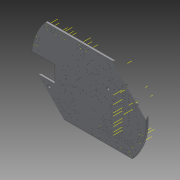
# Autodesk Inventor part: pcb
Saved by Autodesk Inventor 2014 (Build 180170000, 170)
## iProperties
Created: 2013-08-24
Part Number: pcb
Material: Generisch
Document SubType Name: Modeling
Designer: Felix
Density: 1 g/cm^3
Appearance: Vorgabe
Mass: 12.5632 g
Surface Area: 148.317 cm^2
Volume: 12.5632 cm^3
Author: Felix
Autodesk Inventor part; units mm, degrees
ref_plane "YZ Plane" through (0, 0, 0) normal (1, 0, 0) x (0, 1, 0)
ref_plane "XZ Plane" through (0, 0, 0) normal (0, 1, 0) x (-1, 0, 0)
ref_plane "XY Plane" through (0, 0, 0) normal (0, 0, 1) x (1, 0, 0)
sketch "Skizze6" plane through (0, 0, 0) normal (0, 1, 0) x (-1, 0, 0)
  circle A0 centre (10.255, 9.23) radius 0.75
  circle A1 centre (17.67, 60.315) radius 0.75
  circle A2 centre (7.87, 44.425) radius 0.75
  circle A3 centre (17.77, 43.405) radius 0.75
  arc A4 (101.2213, 24.5689) -> (101.2218, 24.5688) centre (101.22155, 24.56885) ccw
  circle A5 centre (77.705, 71.07) radius 0.75
  circle A6 centre (11.055, 72.63) radius 0.75
  circle A7 centre (60.675, 71.27) radius 0.75
  circle A8 centre (78.855, 9.13) radius 0.75
  circle A9 centre (91.045, 71.07) radius 0.75
  circle A10 centre (32.7, 50.6) radius 1.4
  circle A11 centre (87.3, 25.1) radius 1.4
  arc A12 (10.3, 5.7508) -> (10.3, 5.6492) centre (10.3, 5.7) ccw
  arc A13 (91, 5.6492) -> (91, 5.7508) centre (91, 5.7) ccw
  line L0 (10.3, 5.7) -> (91, 5.7)
  arc A14 (10.3, 74.8508) -> (10.3, 74.7492) centre (10.3, 74.8) ccw
  arc A15 (90.6, 74.7492) -> (90.6, 74.8508) centre (90.6, 74.8) ccw
  line L1 (10.3, 74.8) -> (90.6, 74.8)
  arc A16 (91.5301, 73.9834) -> (91.5297, 73.9831) centre (91.5299, 73.98325) ccw
  arc A17 (91.5297, 6.6169) -> (91.5301, 6.6166) centre (91.5299, 6.61675) ccw
  arc A18 (91.5301, 73.9834) -> (91.5297, 73.9831) centre (91.5299, 73.98325) ccw
  arc A19 (101.2213, 24.5689) -> (101.2218, 24.5688) centre (101.22155, 24.56885) ccw
  arc A20 (101.2218, 24.5688) -> (101.2213, 24.5689) centre (101.22155, 24.56885) ccw
  arc A21 (91.5297, 6.6169) -> (91.5301, 6.6166) centre (91.5299, 6.61675) ccw
  arc A22 (91.5299, 6.6167) -> (101.2216, 24.5689) centre (50.590633, 40.310418) ccw
  arc A23 (91.5301, 73.9834) -> (91.5297, 73.9831) centre (91.5299, 73.98325) ccw
  arc A24 (101.2213, 56.0311) -> (101.2218, 56.0312) centre (101.22155, 56.03115) ccw
  arc A25 (101.2216, 56.0312) -> (91.5299, 73.9833) centre (50.590888, 40.289632) ccw
  arc A26 (101.2218, 56.0312) -> (101.2213, 56.0311) centre (101.22155, 56.03115) ccw
  arc A27 (101.2213, 24.5689) -> (101.2218, 24.5688) centre (101.22155, 24.56885) ccw
  arc A28 (91.5301, 73.9834) -> (91.5297, 73.9831) centre (91.5299, 73.98325) ccw
  arc A29 (101.2213, 56.0311) -> (101.2218, 56.0312) centre (101.22155, 56.03115) ccw
  arc A30 (101.2216, 56.0312) -> (91.5299, 73.9833) centre (50.590888, 40.289632) ccw
  arc A31 (101.2218, 56.0312) -> (101.2213, 56.0311) centre (101.22155, 56.03115) ccw
  arc A32 (101.2213, 24.5689) -> (101.2218, 24.5688) centre (101.22155, 24.56885) ccw
  arc A33 (101.2218, 24.5688) -> (101.2213, 24.5689) centre (101.22155, 24.56885) ccw
  arc A34 (91.5297, 6.6169) -> (91.5301, 6.6166) centre (91.5299, 6.61675) ccw
  arc A35 (91.5299, 6.6167) -> (101.2216, 24.5689) centre (50.590633, 40.310418) ccw
  arc A36 (91.5301, 73.9834) -> (91.5297, 73.9831) centre (91.5299, 73.98325) ccw
  arc A37 (101.2213, 56.0311) -> (101.2218, 56.0312) centre (101.22155, 56.03115) ccw
  arc A38 (101.2216, 56.0312) -> (91.5299, 73.9833) centre (50.590888, 40.289632) ccw
  arc A39 (101.2218, 56.0312) -> (101.2213, 56.0311) centre (101.22155, 56.03115) ccw
  arc A40 (101.2213, 24.5689) -> (101.2218, 24.5688) centre (101.22155, 24.56885) ccw
  arc A41 (101.2218, 24.5688) -> (101.2213, 24.5689) centre (101.22155, 24.56885) ccw
  arc A42 (91.5297, 6.6169) -> (91.5301, 6.6166) centre (91.5299, 6.61675) ccw
  arc A43 (91.5299, 6.6167) -> (101.2216, 24.5689) centre (50.590633, 40.310418) ccw
  arc A44 (91.5301, 73.9834) -> (91.5297, 73.9831) centre (91.5299, 73.98325) ccw
  arc A45 (101.2213, 56.0311) -> (101.2218, 56.0312) centre (101.22155, 56.03115) ccw
  arc A46 (101.2216, 56.0312) -> (91.5299, 73.9833) centre (50.590888, 40.289632) ccw
  arc A47 (101.2218, 56.0312) -> (101.2213, 56.0311) centre (101.22155, 56.03115) ccw
  arc A48 (101.2213, 24.5689) -> (101.2218, 24.5688) centre (101.22155, 24.56885) ccw
  arc A49 (101.2218, 24.5688) -> (101.2213, 24.5689) centre (101.22155, 24.56885) ccw
  arc A50 (91.5297, 6.6169) -> (91.5301, 6.6166) centre (91.5299, 6.61675) ccw
  arc A51 (91.5299, 6.6167) -> (101.2216, 24.5689) centre (50.590633, 40.310418) ccw
  arc A52 (91.5301, 73.9834) -> (91.5297, 73.9831) centre (91.5299, 73.98325) ccw
  arc A53 (101.2213, 56.0311) -> (101.2218, 56.0312) centre (101.22155, 56.03115) ccw
  arc A54 (101.2216, 56.0312) -> (91.5299, 73.9833) centre (50.590888, 40.289632) ccw
  arc A55 (101.2218, 56.0312) -> (101.2213, 56.0311) centre (101.22155, 56.03115) ccw
  arc A56 (101.2213, 24.5689) -> (101.2218, 24.5688) centre (101.22155, 24.56885) ccw
  arc A57 (101.2218, 24.5688) -> (101.2213, 24.5689) centre (101.22155, 24.56885) ccw
  arc A58 (91.5297, 6.6169) -> (91.5301, 6.6166) centre (91.5299, 6.61675) ccw
  arc A59 (91.5299, 6.6167) -> (101.2216, 24.5689) centre (50.590633, 40.310418) ccw
  arc A60 (98.4945, 63.0178) -> (98.4941, 63.0176) centre (98.4943, 63.0177) ccw
  arc A61 (101.2213, 56.0311) -> (101.2218, 56.0312) centre (101.22155, 56.03115) ccw
  arc A62 (101.2216, 56.0312) -> (98.4943, 63.0177) centre (50.580091, 40.287993) ccw
  arc A63 (91.5301, 73.9834) -> (91.5297, 73.9831) centre (91.5299, 73.98325) ccw
  arc A64 (98.4941, 63.0176) -> (98.4945, 63.0178) centre (98.4943, 63.0177) ccw
  arc A65 (98.4943, 63.0177) -> (91.5299, 73.9833) centre (50.605086, 40.297009) ccw
  arc A66 (98.4945, 63.0178) -> (98.4941, 63.0176) centre (98.4943, 63.0177) ccw
  arc A67 (101.2213, 56.0311) -> (101.2218, 56.0312) centre (101.22155, 56.03115) ccw
  arc A68 (101.2216, 56.0312) -> (98.4943, 63.0177) centre (50.580091, 40.287993) ccw
  arc A69 (101.2218, 56.0312) -> (101.2213, 56.0311) centre (101.22155, 56.03115) ccw
  arc A70 (101.2213, 24.5689) -> (101.2218, 24.5688) centre (101.22155, 24.56885) ccw
  arc A71 (101.2218, 24.5688) -> (101.2213, 24.5689) centre (101.22155, 24.56885) ccw
  arc A72 (91.5297, 6.6169) -> (91.5301, 6.6166) centre (91.5299, 6.61675) ccw
  arc A73 (91.5299, 6.6167) -> (101.2216, 24.5689) centre (50.590633, 40.310418) ccw
  arc A74 (9.6899, 6.6166) -> (9.6903, 6.6169) centre (9.6901, 6.61675) ccw
  arc A75 (9.6903, 73.9831) -> (9.6899, 73.9834) centre (9.6901, 73.98325) ccw
  arc A76 (9.6901, 73.9833) -> (9.6901, 6.6167) centre (50.615687, 40.3) ccw
  arc A77 (9.6899, 6.6166) -> (9.6903, 6.6169) centre (9.6901, 6.61675) ccw
  arc A78 (9.6903, 73.9831) -> (9.6899, 73.9834) centre (9.6901, 73.98325) ccw
  arc A79 (9.6901, 73.9833) -> (9.6901, 6.6167) centre (50.615687, 40.3) ccw
  arc A80 (9.6899, 6.6166) -> (9.6903, 6.6169) centre (9.6901, 6.61675) ccw
  arc A81 (9.6903, 73.9831) -> (9.6899, 73.9834) centre (9.6901, 73.98325) ccw
  arc A82 (9.6901, 73.9833) -> (9.6901, 6.6167) centre (50.615687, 40.3) ccw
  arc A83 (9.6899, 6.6166) -> (9.6903, 6.6169) centre (9.6901, 6.61675) ccw
  arc A84 (9.6903, 73.9831) -> (9.6899, 73.9834) centre (9.6901, 73.98325) ccw
  arc A85 (9.6901, 73.9833) -> (9.6901, 6.6167) centre (50.615687, 40.3) ccw
  arc A86 (9.6899, 6.6166) -> (9.6903, 6.6169) centre (9.6901, 6.61675) ccw
  arc A87 (9.6903, 73.9831) -> (9.6899, 73.9834) centre (9.6901, 73.98325) ccw
  arc A88 (9.6901, 73.9833) -> (9.6901, 6.6167) centre (50.615687, 40.3) ccw
  arc A89 (9.6899, 6.6166) -> (9.6903, 6.6169) centre (9.6901, 6.61675) ccw
  arc A90 (9.6903, 73.9831) -> (9.6899, 73.9834) centre (9.6901, 73.98325) ccw
  arc A91 (9.6901, 73.9833) -> (9.6901, 6.6167) centre (50.615687, 40.3) ccw
  arc A92 (9.6899, 6.6166) -> (9.6903, 6.6169) centre (9.6901, 6.61675) ccw
  arc A93 (9.6903, 73.9831) -> (9.6899, 73.9834) centre (9.6901, 73.98325) ccw
  arc A94 (9.6901, 73.9833) -> (9.6901, 6.6167) centre (50.615687, 40.3) ccw
  arc A95 (9.6899, 6.6166) -> (9.6903, 6.6169) centre (9.6901, 6.61675) ccw
  arc A96 (9.6903, 73.9831) -> (9.6899, 73.9834) centre (9.6901, 73.98325) ccw
  arc A97 (9.6901, 73.9833) -> (9.6901, 6.6167) centre (50.615687, 40.3) ccw
  arc A98 (9.6899, 6.6166) -> (9.6903, 6.6169) centre (9.6901, 6.61675) ccw
  arc A99 (9.6903, 73.9831) -> (9.6899, 73.9834) centre (9.6901, 73.98325) ccw
  arc A100 (9.6901, 73.9833) -> (9.6901, 6.6167) centre (50.615687, 40.3) ccw
  arc A101 (91.5301, 73.9834) -> (91.5297, 73.9831) centre (91.5299, 73.98325) ccw
  arc A102 (98.4941, 63.0176) -> (98.4945, 63.0178) centre (98.4943, 63.0177) ccw
  arc A103 (98.4943, 63.0177) -> (91.5299, 73.9833) centre (50.605086, 40.297009) ccw
  arc A104 (98.4945, 63.0178) -> (98.4941, 63.0176) centre (98.4943, 63.0177) ccw
  arc A105 (101.2213, 56.0311) -> (101.2218, 56.0312) centre (101.22155, 56.03115) ccw
  arc A106 (101.2216, 56.0312) -> (98.4943, 63.0177) centre (50.580091, 40.287993) ccw
  arc A107 (101.2218, 56.0312) -> (101.2213, 56.0311) centre (101.22155, 56.03115) ccw
  arc A108 (101.2218, 24.5688) -> (101.2213, 24.5689) centre (101.22155, 24.56885) ccw
  arc A109 (91.5297, 6.6169) -> (91.5301, 6.6166) centre (91.5299, 6.61675) ccw
  arc A110 (91.5299, 6.6167) -> (101.2216, 24.5689) centre (50.590633, 40.310418) ccw
  arc A111 (91.5301, 73.9834) -> (91.5297, 73.9831) centre (91.5299, 73.98325) ccw
  arc A112 (98.4941, 63.0176) -> (98.4945, 63.0178) centre (98.4943, 63.0177) ccw
  arc A113 (98.4943, 63.0177) -> (91.5299, 73.9833) centre (50.605086, 40.297009) ccw
  arc A114 (98.4945, 63.0178) -> (98.4941, 63.0176) centre (98.4943, 63.0177) ccw
  arc A115 (101.2213, 56.0311) -> (101.2218, 56.0312) centre (101.22155, 56.03115) ccw
  arc A116 (101.2216, 56.0312) -> (98.4943, 63.0177) centre (50.580091, 40.287993) ccw
  arc A117 (101.2218, 56.0312) -> (101.2213, 56.0311) centre (101.22155, 56.03115) ccw
  arc A118 (101.2213, 24.5689) -> (101.2218, 24.5688) centre (101.22155, 24.56885) ccw
  arc A119 (101.2218, 24.5688) -> (101.2213, 24.5689) centre (101.22155, 24.56885) ccw
  arc A120 (91.5297, 6.6169) -> (91.5301, 6.6166) centre (91.5299, 6.61675) ccw
  arc A121 (91.5299, 6.6167) -> (101.2216, 24.5689) centre (50.590633, 40.310418) ccw
  arc A122 (98.4945, 63.0178) -> (98.4941, 63.0176) centre (98.4943, 63.0177) ccw
  arc A123 (101.2213, 56.0311) -> (101.2218, 56.0312) centre (101.22155, 56.03115) ccw
  arc A124 (101.2216, 56.0312) -> (98.4943, 63.0177) centre (50.580091, 40.287993) ccw
  arc A125 (91.5301, 73.9834) -> (91.5297, 73.9831) centre (91.5299, 73.98325) ccw
  arc A126 (98.4941, 63.0176) -> (98.4945, 63.0178) centre (98.4943, 63.0177) ccw
  arc A127 (98.4943, 63.0177) -> (91.5299, 73.9833) centre (50.605086, 40.297009) ccw
  arc A128 (98.4945, 63.0178) -> (98.4941, 63.0176) centre (98.4943, 63.0177) ccw
  arc A129 (101.2213, 56.0311) -> (101.2218, 56.0312) centre (101.22155, 56.03115) ccw
  arc A130 (101.2216, 56.0312) -> (98.4943, 63.0177) centre (50.580091, 40.287993) ccw
  arc A131 (101.2218, 56.0312) -> (101.2213, 56.0311) centre (101.22155, 56.03115) ccw
  arc A132 (98.4941, 17.5824) -> (98.4945, 17.5822) centre (98.4943, 17.5823) ccw
  arc A133 (98.4945, 17.5822) -> (98.4941, 17.5824) centre (98.4943, 17.5823) ccw
  arc A134 (91.5297, 6.6169) -> (91.5301, 6.6166) centre (91.5299, 6.61675) ccw
  arc A135 (91.5299, 6.6167) -> (98.4943, 17.5823) centre (50.605086, 40.302991) ccw
  arc A136 (91.5301, 73.9834) -> (91.5297, 73.9831) centre (91.5299, 73.98325) ccw
  arc A137 (98.4941, 63.0176) -> (98.4945, 63.0178) centre (98.4943, 63.0177) ccw
  arc A138 (98.4943, 63.0177) -> (91.5299, 73.9833) centre (50.605086, 40.297009) ccw
  arc A139 (98.4945, 63.0178) -> (98.4941, 63.0176) centre (98.4943, 63.0177) ccw
  arc A140 (101.2213, 56.0311) -> (101.2218, 56.0312) centre (101.22155, 56.03115) ccw
  arc A141 (101.2216, 56.0312) -> (98.4943, 63.0177) centre (50.580091, 40.287993) ccw
  arc A142 (101.2218, 56.0312) -> (101.2213, 56.0311) centre (101.22155, 56.03115) ccw
  arc A143 (98.4941, 17.5824) -> (98.4945, 17.5822) centre (98.4943, 17.5823) ccw
  arc A144 (98.4945, 17.5822) -> (98.4941, 17.5824) centre (98.4943, 17.5823) ccw
  arc A145 (91.5297, 6.6169) -> (91.5301, 6.6166) centre (91.5299, 6.61675) ccw
  arc A146 (91.5299, 6.6167) -> (98.4943, 17.5823) centre (50.605086, 40.302991) ccw
  arc A147 (91.5301, 73.9834) -> (91.5297, 73.9831) centre (91.5299, 73.98325) ccw
  arc A148 (98.4941, 63.0176) -> (98.4945, 63.0178) centre (98.4943, 63.0177) ccw
  arc A149 (98.4943, 63.0177) -> (91.5299, 73.9833) centre (50.605086, 40.297009) ccw
  arc A150 (98.4945, 63.0178) -> (98.4941, 63.0176) centre (98.4943, 63.0177) ccw
  arc A151 (101.2213, 56.0311) -> (101.2218, 56.0312) centre (101.22155, 56.03115) ccw
  arc A152 (101.2216, 56.0312) -> (98.4943, 63.0177) centre (50.580091, 40.287993) ccw
  arc A153 (101.2218, 56.0312) -> (101.2213, 56.0311) centre (101.22155, 56.03115) ccw
  arc A154 (98.4941, 17.5824) -> (98.4945, 17.5822) centre (98.4943, 17.5823) ccw
  arc A155 (98.4945, 17.5822) -> (98.4941, 17.5824) centre (98.4943, 17.5823) ccw
  arc A156 (91.5297, 6.6169) -> (91.5301, 6.6166) centre (91.5299, 6.61675) ccw
  arc A157 (91.5299, 6.6167) -> (98.4943, 17.5823) centre (50.605086, 40.302991) ccw
  arc A158 (91.5301, 73.9834) -> (91.5297, 73.9831) centre (91.5299, 73.98325) ccw
  arc A159 (98.4941, 63.0176) -> (98.4945, 63.0178) centre (98.4943, 63.0177) ccw
  arc A160 (98.4943, 63.0177) -> (91.5299, 73.9833) centre (50.605086, 40.297009) ccw
  arc A161 (98.4945, 63.0178) -> (98.4941, 63.0176) centre (98.4943, 63.0177) ccw
  arc A162 (101.2213, 56.0311) -> (101.2218, 56.0312) centre (101.22155, 56.03115) ccw
  arc A163 (101.2216, 56.0312) -> (98.4943, 63.0177) centre (50.580091, 40.287993) ccw
  arc A164 (101.2218, 56.0312) -> (101.2213, 56.0311) centre (101.22155, 56.03115) ccw
  arc A165 (98.4941, 17.5824) -> (98.4945, 17.5822) centre (98.4943, 17.5823) ccw
  arc A166 (98.4945, 17.5822) -> (98.4941, 17.5824) centre (98.4943, 17.5823) ccw
  arc A167 (91.5297, 6.6169) -> (91.5301, 6.6166) centre (91.5299, 6.61675) ccw
  arc A168 (91.5299, 6.6167) -> (98.4943, 17.5823) centre (50.605086, 40.302991) ccw
  circle A169 centre (10.4, 20.5) radius 0.254
  circle A170 centre (23.03, 70.23) radius 0.254
  circle A171 centre (31.4, 70.3) radius 0.254
  circle A172 centre (40.4, 42.8) radius 0.254
  circle A173 centre (22.7, 43.5) radius 0.254
  circle A174 centre (20, 45) radius 0.254
  circle A175 centre (58.2, 64.5) radius 0.254
  circle A176 centre (65.6, 60.7) radius 0.254
  circle A177 centre (55.6, 63.3) radius 0.254
  circle A178 centre (46.2, 27.8) radius 0.254
  circle A179 centre (42.8, 57) radius 0.254
  circle A180 centre (61, 69.2) radius 0.254
  circle A181 centre (50.1, 53.6) radius 0.254
  circle A182 centre (52.4, 53.6) radius 0.254
  circle A183 centre (41.2, 60) radius 0.254
  circle A184 centre (48.8, 39.9) radius 0.254
  circle A185 centre (44.1, 39.8) radius 0.254
  circle A186 centre (30.1, 39.4) radius 0.254
  circle A187 centre (37.1, 13.3) radius 0.254
  circle A188 centre (33.2, 13.3) radius 0.254
  circle A189 centre (76.305, 72.87) radius 0.4064
  circle A190 centre (75.035, 70.33) radius 0.4064
  circle A191 centre (73.765, 72.87) radius 0.4064
  circle A192 centre (72.495, 70.33) radius 0.4064
  circle A193 centre (19.57, 42.005) radius 0.4064
  circle A194 centre (17.03, 40.735) radius 0.4064
  circle A195 centre (19.57, 39.465) radius 0.4064
  circle A196 centre (17.03, 38.195) radius 0.4064
  circle A197 centre (19.47, 58.915) radius 0.4064
  circle A198 centre (16.93, 57.645) radius 0.4064
  circle A199 centre (19.47, 56.375) radius 0.4064
  circle A200 centre (16.93, 55.105) radius 0.4064
  circle A201 centre (19.47, 53.835) radius 0.4064
  circle A202 centre (16.93, 52.565) radius 0.4064
  circle A203 centre (19.47, 51.295) radius 0.4064
  circle A204 centre (16.93, 50.025) radius 0.4064
  circle A205 centre (19.47, 48.755) radius 0.4064
  circle A206 centre (16.93, 47.485) radius 0.4064
  circle A207 centre (9.67, 45.825) radius 0.4064
  circle A208 centre (7.13, 47.095) radius 0.4064
  circle A209 centre (9.67, 48.365) radius 0.4064
  circle A210 centre (7.13, 49.635) radius 0.4064
  circle A211 centre (9.67, 50.905) radius 0.4064
  circle A212 centre (7.13, 52.175) radius 0.4064
  circle A213 centre (12.455, 70.83) radius 0.4064
  circle A214 centre (13.725, 73.37) radius 0.4064
  circle A215 centre (14.995, 70.83) radius 0.4064
  circle A216 centre (16.265, 73.37) radius 0.4064
  circle A217 centre (17.535, 70.83) radius 0.4064
  circle A218 centre (18.805, 73.37) radius 0.4064
  circle A219 centre (20.075, 70.83) radius 0.4064
  circle A220 centre (21.345, 73.37) radius 0.4064
  circle A221 centre (11.655, 7.43) radius 0.4064
  circle A222 centre (12.925, 9.97) radius 0.4064
  circle A223 centre (14.195, 7.43) radius 0.4064
  circle A224 centre (15.465, 9.97) radius 0.4064
  circle A225 centre (16.735, 7.43) radius 0.4064
  circle A226 centre (18.005, 9.97) radius 0.4064
  circle A227 centre (19.275, 7.43) radius 0.4064
  circle A228 centre (20.545, 9.97) radius 0.4064
  circle A229 centre (4.9078, 62.6827) radius 0.4064
  circle A230 centre (6.7307, 60.5053) radius 0.4064
  circle A231 centre (3.895, 60.3534) radius 0.4064
  circle A232 centre (5.7179, 58.1759) radius 0.4064
  circle A233 centre (2.8821, 58.0241) radius 0.4064
  circle A234 centre (4.705, 55.8466) radius 0.4064
  circle A235 centre (1.8693, 55.6947) radius 0.4064
  circle A236 centre (3.6922, 53.5173) radius 0.4064
  circle A237 centre (0.3852, 29.2123) radius 0.4064
  circle A238 centre (3.1969, 28.8139) radius 0.4064
  circle A239 centre (1.1912, 26.8036) radius 0.4064
  circle A240 centre (4.0029, 26.4052) radius 0.4064
  circle A241 centre (1.9971, 24.3948) radius 0.4064
  circle A242 centre (4.8088, 23.9964) radius 0.4064
  circle A243 centre (2.8031, 21.9861) radius 0.4064
  circle A244 centre (5.6148, 21.5877) radius 0.4064
  circle A245 centre (59.275, 73.07) radius 0.4064
  circle A246 centre (64.6, 17.4) radius 0.254
  circle A247 centre (56.735, 73.07) radius 0.4064
  circle A248 centre (55.465, 70.53) radius 0.4064
  circle A249 centre (54.195, 73.07) radius 0.4064
  circle A250 centre (52.925, 70.53) radius 0.4064
  circle A251 centre (60.3, 44.5) radius 0.254
  circle A252 centre (80.255, 7.33) radius 0.4064
  circle A253 centre (81.525, 9.87) radius 0.4064
  circle A254 centre (82.795, 7.33) radius 0.4064
  circle A255 centre (84.065, 9.87) radius 0.4064
  circle A256 centre (85.335, 7.33) radius 0.4064
  circle A257 centre (86.605, 9.87) radius 0.4064
  circle A258 centre (87.875, 7.33) radius 0.4064
  circle A259 centre (89.145, 9.87) radius 0.4064
  circle A260 centre (64, 36.4) radius 0.254
  circle A261 centre (89.645, 72.87) radius 0.4064
  circle A262 centre (88.375, 70.33) radius 0.4064
  circle A263 centre (87.105, 72.87) radius 0.4064
  circle A264 centre (85.835, 70.33) radius 0.4064
  circle A265 centre (84.565, 72.87) radius 0.4064
  circle A266 centre (83.295, 70.33) radius 0.4064
  circle A267 centre (82.025, 72.87) radius 0.4064
  circle A268 centre (80.755, 70.33) radius 0.4064
  circle A269 centre (71.9, 28.8) radius 0.254
  circle A270 centre (96.5044, 17.5038) radius 0.4064
  circle A271 centre (94.6288, 19.6361) radius 0.4064
  circle A272 centre (97.46, 19.8572) radius 0.4064
  circle A273 centre (95.5844, 21.9895) radius 0.4064
  circle A274 centre (98.4156, 22.2105) radius 0.4064
  circle A275 centre (96.54, 24.3428) radius 0.4064
  circle A276 centre (99.3712, 24.5639) radius 0.4064
  circle A277 centre (97.4956, 26.6962) radius 0.4064
  circle A278 centre (101.1281, 52.2968) radius 0.4064
  circle A279 centre (98.315, 52.6854) radius 0.4064
  circle A280 centre (100.3137, 54.7027) radius 0.4064
  circle A281 centre (97.5006, 55.0913) radius 0.4064
  circle A282 centre (99.4994, 57.1087) radius 0.4064
  circle A283 centre (96.6863, 57.4973) radius 0.4064
  circle A284 centre (98.685, 59.5146) radius 0.4064
  circle A285 centre (95.8719, 59.9032) radius 0.4064
  circle A286 centre (59.2, 45.4) radius 0.254
  circle A287 centre (62.7, 37) radius 0.254
  circle A288 centre (40.6488, 11.4606) radius 0.508
  circle A289 centre (47.1512, 11.4606) radius 0.508
  circle A290 centre (40.6488, 6.9394) radius 0.508
  circle A291 centre (47.1512, 6.9394) radius 0.508
  circle A292 centre (60.2, 55.087) radius 0.4064
  circle A293 centre (60.2, 59.913) radius 0.4064
  circle A294 centre (19.43, 33.62) radius 0.508
  circle A295 centre (19.43, 31.08) radius 0.508
  circle A296 centre (19.47, 21.59) radius 0.508
  circle A297 centre (19.47, 24.13) radius 0.508
  circle A298 centre (19.47, 26.67) radius 0.508
  circle A299 centre (35.032, 15.304) radius 0.508
  circle A300 centre (29.952, 15.304) radius 0.508
  circle A301 centre (27.412, 15.304) radius 0.508
  circle A302 centre (27.412, 17.844) radius 0.508
  circle A303 centre (24.872, 17.844) radius 0.508
  circle A304 centre (22.332, 15.304) radius 0.508
  circle A305 centre (22.332, 17.844) radius 0.508
  circle A306 centre (19.792, 15.304) radius 0.508
  circle A307 centre (17.252, 15.304) radius 0.508
  circle A308 centre (37.572, 17.844) radius 0.508
  circle A309 centre (32.492, 17.844) radius 0.508
  circle A310 centre (35.032, 17.844) radius 0.508
  circle A311 centre (37.572, 15.304) radius 0.508
  circle A312 centre (40.112, 15.304) radius 0.508
  circle A313 centre (17.252, 17.844) radius 0.508
  circle A314 centre (14.712, 17.844) radius 0.508
  circle A315 centre (12.172, 17.844) radius 0.508
  circle A316 centre (32.492, 15.304) radius 0.508
  circle A317 centre (24.872, 15.304) radius 0.508
  circle A318 centre (14.712, 15.304) radius 0.508
  circle A319 centre (40.112, 17.844) radius 0.508
  circle A320 centre (19.792, 17.844) radius 0.508
  circle A321 centre (12.172, 15.304) radius 0.508
  circle A322 centre (9.632, 15.304) radius 0.508
  circle A323 centre (29.952, 17.844) radius 0.508
  circle A324 centre (9.632, 17.844) radius 0.508
  circle A325 centre (13.4, 54.57) radius 0.508
  circle A326 centre (13.4, 44.41) radius 0.508
  circle A327 centre (13.4, 46.95) radius 0.508
  circle A328 centre (13.4, 34.25) radius 0.508
  circle A329 centre (13.4, 31.71) radius 0.508
  circle A330 centre (13.4, 41.87) radius 0.508
  circle A331 centre (13.4, 36.79) radius 0.508
  circle A332 centre (13.4, 49.49) radius 0.508
  circle A333 centre (13.4, 39.33) radius 0.508
  circle A334 centre (13.4, 52.03) radius 0.508
  circle A335 centre (67.5, 21.8) radius 0.254
  circle A336 centre (29.3, 57.4) radius 0.254
  circle A337 centre (25.4, 47.4) radius 0.254
  circle A338 centre (30.4, 58.3) radius 0.254
  circle A339 centre (26.6, 44.3) radius 0.254
  circle A340 centre (27.1, 52.8) radius 0.254
  circle A341 centre (27.4, 43.2) radius 0.254
  circle A342 centre (27, 40) radius 0.254
  circle A343 centre (29.2, 25.3) radius 0.254
  circle A344 centre (36.9, 52.1) radius 0.254
  circle A345 centre (36, 42.7) radius 0.254
  circle A346 centre (29.7, 32.3) radius 0.254
  circle A347 centre (29.8, 27.1) radius 0.254
  circle A348 centre (32.9, 25.7) radius 0.254
  circle A349 centre (36.5, 57.8) radius 0.254
  circle A350 centre (41.7, 37.3) radius 0.254
  circle A351 centre (42.4, 39.8) radius 0.254
  circle A352 centre (42, 14.1) radius 0.254
  circle A353 centre (51.8, 60.7) radius 0.254
  circle A354 centre (52.1, 55.5) radius 0.254
  circle A355 centre (52.9, 56.8) radius 0.254
  circle A356 centre (55.6, 64.7) radius 0.254
  circle A357 centre (54.6, 67.8) radius 0.254
  circle A358 centre (73.4, 19.4) radius 0.254
  circle A359 centre (78.1, 19.4) radius 0.254
  circle A360 centre (77.4, 16.7) radius 0.254
  circle A361 centre (69.7, 16.8) radius 0.254
  circle A362 centre (77.3, 24.7) radius 0.254
  circle A363 centre (72.9, 27.3) radius 0.254
  circle A364 centre (26.8, 57.4) radius 0.254
  circle A365 centre (30.1, 38) radius 0.254
  circle A366 centre (31.6, 59.4) radius 0.254
  circle A367 centre (27.7, 33) radius 0.254
  circle A368 centre (28.8, 43.2) radius 0.254
  circle A369 centre (30.3, 34.6) radius 0.254
  circle A370 centre (34, 41.7) radius 0.254
  circle A371 centre (32.2, 57.4) radius 0.254
  circle A372 centre (70.6, 42.4) radius 0.254
  circle A373 centre (24.5, 72.5) radius 0.254
  circle A374 centre (71.1, 39.3) radius 0.254
  circle A375 centre (11.2, 60.8) radius 0.254
  circle A376 centre (22.2, 27.1) radius 0.254
  circle A377 centre (72.3, 38.7) radius 0.254
  circle A378 centre (38.7, 23.6) radius 0.254
  circle A379 centre (76, 14.9) radius 0.254
  circle A380 centre (34, 19.5) radius 0.254
  circle A381 centre (75.2, 44) radius 0.254
  circle A382 centre (76.7, 10.1) radius 0.254
  circle A383 centre (10.5, 64.9) radius 0.254
  circle A384 centre (4.7, 37.2) radius 0.254
  circle A385 centre (92.4, 26.6) radius 0.254
  circle A386 centre (62.5, 17.2) radius 0.254
  circle A387 centre (82.8, 17.4) radius 0.254
  circle A388 centre (67.8, 12.5) radius 0.254
  circle A389 centre (37.3, 21) radius 0.254
  circle A390 centre (82.7, 11.6) radius 0.254
  circle A391 centre (8.4, 63) radius 0.254
  circle A392 centre (30, 65.2) radius 0.254
  circle A393 centre (43.5, 43.1) radius 0.254
  circle A394 centre (5.7, 35.9) radius 0.254
  circle A395 centre (7.5, 13.7) radius 0.254
  circle A396 centre (36.7, 23.3) radius 0.254
  circle A397 centre (3.3, 30.6) radius 0.254
  circle A398 centre (69.1, 12.5) radius 0.254
  circle A399 centre (90.2, 17.7) radius 0.254
  circle A400 centre (13.1, 67.2) radius 0.254
  circle A401 centre (11.7, 68.6) radius 0.254
  circle A402 centre (31, 67.1) radius 0.254
  circle A403 centre (43.6, 44.9) radius 0.254
  circle A404 centre (11.5, 12.1) radius 0.254
  circle A405 centre (70, 9) radius 0.254
  circle A406 centre (35.2, 22.6) radius 0.254
  circle A407 centre (90.1, 19.2) radius 0.254
  circle A408 centre (63.5, 15.5) radius 0.254
  circle A409 centre (14.7, 68.1) radius 0.254
  circle A410 centre (29.86, 68.94) radius 0.254
  circle A411 centre (42, 45) radius 0.254
  circle A412 centre (56, 36.9) radius 0.254
  circle A413 centre (37, 26.4) radius 0.254
  circle A414 centre (31.4, 25.7) radius 0.254
  circle A415 centre (63.5, 21.7) radius 0.254
  circle A416 centre (11.2, 59.3) radius 0.254
  circle A417 centre (23.7, 27.1) radius 0.254
  circle A418 centre (64.7, 24.4) radius 0.254
  circle A419 centre (35.6, 24.7) radius 0.254
  circle A420 centre (30.6, 23.7) radius 0.254
  circle A421 centre (65.5, 26.3) radius 0.254
  circle A422 centre (66.6, 29.3) radius 0.254
  circle A423 centre (79.7, 15.9) radius 0.254
  circle A424 centre (67.7, 30.3) radius 0.254
  circle A425 centre (97.8, 48.7) radius 0.254
  circle A426 centre (76.2, 31.4) radius 0.254
  circle A427 centre (74.1, 33.1) radius 0.254
  circle A428 centre (32.9, 70.3) radius 0.254
  circle A429 centre (26.85, 36.1) radius 0.254
  circle A430 centre (31.7, 12.5) radius 0.254
  circle A431 centre (12.6, 63.9) radius 0.254
  circle A432 centre (67.7, 48.9) radius 0.254
  circle A433 centre (95.9, 49.8) radius 0.254
  circle A434 centre (61.3, 37.9) radius 0.254
  circle A435 centre (62.9, 26.4) radius 0.254
  circle A436 centre (62.4, 47.4) radius 0.254
  circle A437 centre (73.5, 12.3) radius 0.254
  circle A438 centre (48.4, 36.7) radius 0.254
  circle A439 centre (68.9, 35.1) radius 0.254
  circle A440 centre (77.5, 33.9) radius 0.254
  circle A441 centre (43.8, 51.3) radius 0.254
  circle A442 centre (41.5, 57.7) radius 0.254
  circle A443 centre (58.5, 34.2) radius 0.254
  circle A444 centre (39.1, 36.7) radius 0.254
  circle A445 centre (52.7, 36.7) radius 0.254
  circle A446 centre (51.1, 72.8) radius 0.254
  circle A447 centre (31.8, 73.1) radius 0.254
  circle A448 centre (49, 45) radius 0.254
  circle A449 centre (42.2, 49.9) radius 0.254
  circle A450 centre (58.005, 70.53) radius 0.4064
  circle A451 centre (66.8, 10.8) radius 0.254
  circle A452 centre (85.4, 13.4) radius 0.254
  circle A453 centre (21.8, 20.7) radius 0.254
  circle A454 centre (30.2, 36.3) radius 0.254
  circle A455 centre (61.1, 11.6) radius 0.254
  circle A456 centre (34, 8.5) radius 0.254
  circle A457 centre (67.9, 73.5) radius 0.254
  circle A458 centre (42, 72.7) radius 0.254
  circle A459 centre (31.8, 68.1) radius 0.254
  circle A460 centre (44.9, 43.2) radius 0.254
  circle A461 centre (29.6, 29.9) radius 0.254
  circle A462 centre (16.7, 29.4) radius 0.254
  circle A463 centre (12.7, 24.2) radius 0.254
  circle A464 centre (61.3, 43.4) radius 0.254
  circle A465 centre (65, 35.6) radius 0.254
  circle A466 centre (72.1, 30.3) radius 0.254
  circle A467 centre (59, 51) radius 0.254
  circle A468 centre (58.4, 46.9) radius 0.254
  circle A469 centre (79.4, 19.3) radius 0.254
  circle A470 centre (66, 36.9) radius 0.254
  circle A471 centre (46.4, 66.7) radius 0.254
  circle A472 centre (34.6, 72) radius 0.254
  circle A473 centre (28.9, 60) radius 0.254
  circle A474 centre (37, 64.9) radius 0.254
  circle A475 centre (43.5, 60.4) radius 0.254
  circle A476 centre (12.6, 62.1) radius 0.254
  circle A477 centre (40.6, 65.4) radius 0.254
  circle A478 centre (22.5, 55) radius 0.254
  circle A479 centre (14.8, 29.4) radius 0.254
  circle A480 centre (45.1, 60.8) radius 0.254
  circle A481 centre (34.6, 64.8) radius 0.254
  circle A482 centre (48.3, 65.6) radius 0.254
  circle A483 centre (29.3, 22.4) radius 0.254
  circle A484 centre (24.9, 56.5) radius 0.254
  circle A485 centre (25.4, 11.6) radius 0.254
  circle A486 centre (56.2, 38.4) radius 0.3
  circle A487 centre (45.3, 55.9) radius 0.254
  circle A488 centre (64.5, 28.9) radius 0.254
  circle A489 centre (86.9, 14.5) radius 0.254
  circle A490 centre (46.7, 55.9) radius 0.254
  circle A491 centre (71.9, 41.7) radius 0.254
  circle A492 centre (48.2, 55.8) radius 0.254
  circle A493 centre (70, 50.1) radius 0.254
  circle A494 centre (71.8, 46.1) radius 0.254
  circle A495 centre (50.9, 61.6) radius 0.254
  circle A496 centre (6.8, 41.4) radius 0.254
  circle A497 centre (11.3, 26.4) radius 0.254
  circle A498 centre (58.8, 36.9) radius 0.254
  circle A499 centre (55.8, 66.5) radius 0.254
  circle A500 centre (48.5, 18.3) radius 0.254
  circle A501 centre (44.9, 26.2) radius 0.254
  circle A502 centre (72.5, 33.9) radius 0.254
  circle A503 centre (34.6, 29.7) radius 0.254
  circle A504 centre (23.5, 23.3) radius 0.254
  circle A505 centre (21.5, 56.3) radius 0.254
  circle A506 centre (9.1, 53.3) radius 0.254
  circle A507 centre (74.2, 47.9) radius 0.254
  circle A508 centre (75.5, 33.3) radius 0.254
  circle A509 centre (60.3, 17.1) radius 0.254
  circle A510 centre (35.9, 20.5) radius 0.254
  circle A511 centre (32.7, 20.5) radius 0.254
  circle A512 centre (89.105, 14.395) radius 0.254
  circle A513 centre (83.6, 14.3) radius 0.254
  circle A514 centre (74.7, 13.7) radius 0.254
  circle A515 centre (23.9, 7.8) radius 0.254
  circle A516 centre (23.9, 11.6) radius 0.254
  circle A517 centre (5.2, 31.8) radius 0.254
  circle A518 centre (50.605086, 40.302991) radius 53.004272
  line L2 (10.363201, 74.8) -> (90.846971, 74.8)
  line L3 (90.755876, 5.7) -> (10.454297, 5.7)
  line L4 (81.989231, 29.954) -> (81.989231, 45.335)
  line L5 (103.369959, 45.335) -> (81.989231, 45.335)
  line L6 (102.589231, 29.954) -> (81.989231, 29.954)
  point P0 (0, 0)
  dimension "d5" = 106.00854
  dimension "d6" = 20.6
  constraints: 519 centre point, 322 point on circle, 14 end point, 4 point on line, 1 coincident, 1 parallel, 1 perpendicular
  measures "d5" diameter of A518
  measures "d6" distance of L6.start L4.start
sketch "Skizze6 outline for Extrusion2" plane through (0, 0, 0) normal (0, 1, 0) x (-1, 0, 0)
  line L0 (81.989231, 29.954) -> (81.989231, 45.335)
  line L1 (102.589231, 29.954) -> (81.989231, 29.954)
  line L2 (81.989231, 45.335) -> (103.369959, 45.335)
  arc A0 (90.755876, 5.7) -> (102.589231, 29.954) centre (50.605086, 40.302991) ccw
  arc A1 (103.369959, 45.335) -> (90.846971, 74.8) centre (50.605086, 40.302991) ccw
  line L3 (10.454297, 5.7) -> (90.755876, 5.7)
  line L4 (90.846971, 74.8) -> (10.363201, 74.8)
  arc A2 (10.363201, 74.8) -> (10.454297, 5.7) centre (50.605086, 40.302991) ccw
  circle A3 centre (11.655, 7.43) radius 0.4064
  circle A4 centre (10.255, 9.23) radius 0.75
  circle A5 centre (11.5, 12.1) radius 0.254
  circle A6 centre (7.5, 13.7) radius 0.254
  circle A7 centre (14.195, 7.43) radius 0.4064
  circle A8 centre (16.735, 7.43) radius 0.4064
  circle A9 centre (12.925, 9.97) radius 0.4064
  circle A10 centre (15.465, 9.97) radius 0.4064
  circle A11 centre (18.005, 9.97) radius 0.4064
  circle A12 centre (19.275, 7.43) radius 0.4064
  circle A13 centre (23.9, 7.8) radius 0.254
  circle A14 centre (20.545, 9.97) radius 0.4064
  circle A15 centre (23.9, 11.6) radius 0.254
  circle A16 centre (9.632, 15.304) radius 0.508
  circle A17 centre (12.172, 15.304) radius 0.508
  circle A18 centre (9.632, 17.844) radius 0.508
  circle A19 centre (12.172, 17.844) radius 0.508
  circle A20 centre (2.8031, 21.9861) radius 0.4064
  circle A21 centre (5.6148, 21.5877) radius 0.4064
  circle A22 centre (10.4, 20.5) radius 0.254
  circle A23 centre (14.712, 15.304) radius 0.508
  circle A24 centre (17.252, 15.304) radius 0.508
  circle A25 centre (14.712, 17.844) radius 0.508
  circle A26 centre (17.252, 17.844) radius 0.508
  circle A27 centre (19.792, 15.304) radius 0.508
  circle A28 centre (22.332, 15.304) radius 0.508
  circle A29 centre (24.872, 15.304) radius 0.508
  circle A30 centre (19.792, 17.844) radius 0.508
  circle A31 centre (22.332, 17.844) radius 0.508
  circle A32 centre (24.872, 17.844) radius 0.508
  circle A33 centre (21.8, 20.7) radius 0.254
  circle A34 centre (19.47, 21.59) radius 0.508
  circle A35 centre (34, 8.5) radius 0.254
  circle A36 centre (25.4, 11.6) radius 0.254
  circle A37 centre (31.7, 12.5) radius 0.254
  circle A38 centre (33.2, 13.3) radius 0.254
  circle A39 centre (37.1, 13.3) radius 0.254
  circle A40 centre (40.6488, 6.9394) radius 0.508
  circle A41 centre (47.1512, 6.9394) radius 0.508
  circle A42 centre (40.6488, 11.4606) radius 0.508
  circle A43 centre (42, 14.1) radius 0.254
  circle A44 centre (47.1512, 11.4606) radius 0.508
  circle A45 centre (27.412, 15.304) radius 0.508
  circle A46 centre (29.952, 15.304) radius 0.508
  circle A47 centre (27.412, 17.844) radius 0.508
  circle A48 centre (29.952, 17.844) radius 0.508
  circle A49 centre (32.492, 15.304) radius 0.508
  circle A50 centre (35.032, 15.304) radius 0.508
  circle A51 centre (37.572, 15.304) radius 0.508
  circle A52 centre (32.492, 17.844) radius 0.508
  circle A53 centre (35.032, 17.844) radius 0.508
  circle A54 centre (37.572, 17.844) radius 0.508
  circle A55 centre (29.3, 22.4) radius 0.254
  circle A56 centre (34, 19.5) radius 0.254
  circle A57 centre (32.7, 20.5) radius 0.254
  circle A58 centre (35.9, 20.5) radius 0.254
  circle A59 centre (37.3, 21) radius 0.254
  circle A60 centre (35.2, 22.6) radius 0.254
  circle A61 centre (40.112, 15.304) radius 0.508
  circle A62 centre (40.112, 17.844) radius 0.508
  circle A63 centre (48.5, 18.3) radius 0.254
  circle A64 centre (1.9971, 24.3948) radius 0.4064
  circle A65 centre (4.8088, 23.9964) radius 0.4064
  circle A66 centre (1.1912, 26.8036) radius 0.4064
  circle A67 centre (4.0029, 26.4052) radius 0.4064
  circle A68 centre (11.3, 26.4) radius 0.254
  circle A69 centre (0.3852, 29.2123) radius 0.4064
  circle A70 centre (3.1969, 28.8139) radius 0.4064
  circle A71 centre (3.3, 30.6) radius 0.254
  circle A72 centre (12.7, 24.2) radius 0.254
  circle A73 centre (19.47, 24.13) radius 0.508
  circle A74 centre (23.5, 23.3) radius 0.254
  circle A75 centre (19.47, 26.67) radius 0.508
  circle A76 centre (22.2, 27.1) radius 0.254
  circle A77 centre (23.7, 27.1) radius 0.254
  circle A78 centre (14.8, 29.4) radius 0.254
  circle A79 centre (16.7, 29.4) radius 0.254
  circle A80 centre (19.43, 31.08) radius 0.508
  circle A81 centre (5.2, 31.8) radius 0.254
  circle A82 centre (5.7, 35.9) radius 0.254
  circle A83 centre (4.7, 37.2) radius 0.254
  circle A84 centre (13.4, 31.71) radius 0.508
  circle A85 centre (13.4, 34.25) radius 0.508
  circle A86 centre (19.43, 33.62) radius 0.508
  circle A87 centre (13.4, 36.79) radius 0.508
  circle A88 centre (13.4, 39.33) radius 0.508
  circle A89 centre (17.03, 38.195) radius 0.4064
  circle A90 centre (19.57, 39.465) radius 0.4064
  circle A91 centre (30.6, 23.7) radius 0.254
  circle A92 centre (29.2, 25.3) radius 0.254
  circle A93 centre (31.4, 25.7) radius 0.254
  circle A94 centre (29.8, 27.1) radius 0.254
  circle A95 centre (36.7, 23.3) radius 0.254
  circle A96 centre (35.6, 24.7) radius 0.254
  circle A97 centre (32.9, 25.7) radius 0.254
  circle A98 centre (37, 26.4) radius 0.254
  circle A99 centre (29.6, 29.9) radius 0.254
  circle A100 centre (34.6, 29.7) radius 0.254
  circle A101 centre (38.7, 23.6) radius 0.254
  circle A102 centre (44.9, 26.2) radius 0.254
  circle A103 centre (46.2, 27.8) radius 0.254
  circle A104 centre (27.7, 33) radius 0.254
  circle A105 centre (29.7, 32.3) radius 0.254
  circle A106 centre (30.3, 34.6) radius 0.254
  circle A107 centre (26.85, 36.1) radius 0.254
  circle A108 centre (30.2, 36.3) radius 0.254
  circle A109 centre (27, 40) radius 0.254
  circle A110 centre (30.1, 38) radius 0.254
  circle A111 centre (30.1, 39.4) radius 0.254
  circle A112 centre (39.1, 36.7) radius 0.254
  circle A113 centre (41.7, 37.3) radius 0.254
  circle A114 centre (42.4, 39.8) radius 0.254
  circle A115 centre (44.1, 39.8) radius 0.254
  circle A116 centre (48.4, 36.7) radius 0.254
  circle A117 centre (48.8, 39.9) radius 0.254
  circle A118 centre (61.1, 11.6) radius 0.254
  circle A119 centre (70, 9) radius 0.254
  circle A120 centre (66.8, 10.8) radius 0.254
  circle A121 centre (67.8, 12.5) radius 0.254
  circle A122 centre (69.1, 12.5) radius 0.254
  circle A123 centre (73.5, 12.3) radius 0.254
  circle A124 centre (74.7, 13.7) radius 0.254
  circle A125 centre (60.3, 17.1) radius 0.254
  circle A126 centre (62.5, 17.2) radius 0.254
  circle A127 centre (63.5, 15.5) radius 0.254
  circle A128 centre (69.7, 16.8) radius 0.254
  circle A129 centre (64.6, 17.4) radius 0.254
  circle A130 centre (76, 14.9) radius 0.254
  circle A131 centre (63.5, 21.7) radius 0.254
  circle A132 centre (67.5, 21.8) radius 0.254
  circle A133 centre (73.4, 19.4) radius 0.254
  circle A134 centre (80.255, 7.33) radius 0.4064
  circle A135 centre (78.855, 9.13) radius 0.75
  circle A136 centre (76.7, 10.1) radius 0.254
  circle A137 centre (81.525, 9.87) radius 0.4064
  circle A138 centre (82.795, 7.33) radius 0.4064
  circle A139 centre (85.335, 7.33) radius 0.4064
  circle A140 centre (87.875, 7.33) radius 0.4064
  circle A141 centre (84.065, 9.87) radius 0.4064
  circle A142 centre (86.605, 9.87) radius 0.4064
  circle A143 centre (82.7, 11.6) radius 0.254
  circle A144 centre (85.4, 13.4) radius 0.254
  circle A145 centre (83.6, 14.3) radius 0.254
  circle A146 centre (86.9, 14.5) radius 0.254
  circle A147 centre (89.145, 9.87) radius 0.4064
  circle A148 centre (89.105, 14.395) radius 0.254
  circle A149 centre (77.4, 16.7) radius 0.254
  circle A150 centre (79.7, 15.9) radius 0.254
  circle A151 centre (82.8, 17.4) radius 0.254
  circle A152 centre (78.1, 19.4) radius 0.254
  circle A153 centre (79.4, 19.3) radius 0.254
  circle A154 centre (90.2, 17.7) radius 0.254
  circle A155 centre (96.5044, 17.5038) radius 0.4064
  circle A156 centre (90.1, 19.2) radius 0.254
  circle A157 centre (94.6288, 19.6361) radius 0.4064
  circle A158 centre (97.46, 19.8572) radius 0.4064
  circle A159 centre (95.5844, 21.9895) radius 0.4064
  circle A160 centre (98.4156, 22.2105) radius 0.4064
  circle A161 centre (62.9, 26.4) radius 0.254
  circle A162 centre (64.7, 24.4) radius 0.254
  circle A163 centre (65.5, 26.3) radius 0.254
  circle A164 centre (72.9, 27.3) radius 0.254
  circle A165 centre (64.5, 28.9) radius 0.254
  circle A166 centre (66.6, 29.3) radius 0.254
  circle A167 centre (67.7, 30.3) radius 0.254
  circle A168 centre (71.9, 28.8) radius 0.254
  circle A169 centre (72.1, 30.3) radius 0.254
  circle A170 centre (58.5, 34.2) radius 0.254
  circle A171 centre (52.7, 36.7) radius 0.254
  circle A172 centre (56, 36.9) radius 0.254
  circle A173 centre (56.2, 38.4) radius 0.3
  circle A174 centre (58.8, 36.9) radius 0.254
  circle A175 centre (61.3, 37.9) radius 0.254
  circle A176 centre (62.7, 37) radius 0.254
  circle A177 centre (65, 35.6) radius 0.254
  circle A178 centre (68.9, 35.1) radius 0.254
  circle A179 centre (74.1, 33.1) radius 0.254
  circle A180 centre (75.5, 33.3) radius 0.254
  circle A181 centre (72.5, 33.9) radius 0.254
  circle A182 centre (64, 36.4) radius 0.254
  circle A183 centre (66, 36.9) radius 0.254
  circle A184 centre (72.3, 38.7) radius 0.254
  circle A185 centre (71.1, 39.3) radius 0.254
  circle A186 centre (77.3, 24.7) radius 0.254
  circle A187 centre (87.3, 25.1) radius 1.4
  circle A188 centre (76.2, 31.4) radius 0.254
  circle A189 centre (92.4, 26.6) radius 0.254
  circle A190 centre (96.54, 24.3428) radius 0.4064
  circle A191 centre (99.3712, 24.5639) radius 0.4064
  circle A192 centre (97.4956, 26.6962) radius 0.4064
  circle A193 centre (77.5, 33.9) radius 0.254
  circle A194 centre (6.8, 41.4) radius 0.254
  circle A195 centre (7.87, 44.425) radius 0.75
  circle A196 centre (9.67, 45.825) radius 0.4064
  circle A197 centre (7.13, 47.095) radius 0.4064
  circle A198 centre (9.67, 48.365) radius 0.4064
  circle A199 centre (13.4, 41.87) radius 0.508
  circle A200 centre (17.03, 40.735) radius 0.4064
  circle A201 centre (17.77, 43.405) radius 0.75
  circle A202 centre (19.57, 42.005) radius 0.4064
  circle A203 centre (22.7, 43.5) radius 0.254
  circle A204 centre (13.4, 44.41) radius 0.508
  circle A205 centre (13.4, 46.95) radius 0.508
  circle A206 centre (16.93, 47.485) radius 0.4064
  circle A207 centre (20, 45) radius 0.254
  circle A208 centre (7.13, 49.635) radius 0.4064
  circle A209 centre (7.13, 52.175) radius 0.4064
  circle A210 centre (9.67, 50.905) radius 0.4064
  circle A211 centre (3.6922, 53.5173) radius 0.4064
  circle A212 centre (1.8693, 55.6947) radius 0.4064
  circle A213 centre (4.705, 55.8466) radius 0.4064
  circle A214 centre (9.1, 53.3) radius 0.254
  circle A215 centre (13.4, 49.49) radius 0.508
  circle A216 centre (16.93, 50.025) radius 0.4064
  circle A217 centre (13.4, 52.03) radius 0.508
  circle A218 centre (16.93, 52.565) radius 0.4064
  circle A219 centre (19.47, 48.755) radius 0.4064
  circle A220 centre (19.47, 51.295) radius 0.4064
  circle A221 centre (13.4, 54.57) radius 0.508
  circle A222 centre (16.93, 55.105) radius 0.4064
  circle A223 centre (19.47, 53.835) radius 0.4064
  circle A224 centre (19.47, 56.375) radius 0.4064
  circle A225 centre (21.5, 56.3) radius 0.254
  circle A226 centre (22.5, 55) radius 0.254
  circle A227 centre (24.9, 56.5) radius 0.254
  circle A228 centre (27.4, 43.2) radius 0.254
  circle A229 centre (26.6, 44.3) radius 0.254
  circle A230 centre (28.8, 43.2) radius 0.254
  circle A231 centre (34, 41.7) radius 0.254
  circle A232 centre (36, 42.7) radius 0.254
  circle A233 centre (25.4, 47.4) radius 0.254
  circle A234 centre (40.4, 42.8) radius 0.254
  circle A235 centre (43.5, 43.1) radius 0.254
  circle A236 centre (44.9, 43.2) radius 0.254
  circle A237 centre (42, 45) radius 0.254
  circle A238 centre (43.6, 44.9) radius 0.254
  circle A239 centre (49, 45) radius 0.254
  circle A240 centre (32.7, 50.6) radius 1.4
  circle A241 centre (36.9, 52.1) radius 0.254
  circle A242 centre (27.1, 52.8) radius 0.254
  circle A243 centre (42.2, 49.9) radius 0.254
  circle A244 centre (43.8, 51.3) radius 0.254
  circle A245 centre (50.1, 53.6) radius 0.254
  circle A246 centre (45.3, 55.9) radius 0.254
  circle A247 centre (46.7, 55.9) radius 0.254
  circle A248 centre (48.2, 55.8) radius 0.254
  circle A249 centre (2.8821, 58.0241) radius 0.4064
  circle A250 centre (5.7179, 58.1759) radius 0.4064
  circle A251 centre (3.895, 60.3534) radius 0.4064
  circle A252 centre (6.7307, 60.5053) radius 0.4064
  circle A253 centre (11.2, 59.3) radius 0.254
  circle A254 centre (11.2, 60.8) radius 0.254
  circle A255 centre (4.9078, 62.6827) radius 0.4064
  circle A256 centre (8.4, 63) radius 0.254
  circle A257 centre (12.6, 62.1) radius 0.254
  circle A258 centre (12.6, 63.9) radius 0.254
  circle A259 centre (10.5, 64.9) radius 0.254
  circle A260 centre (16.93, 57.645) radius 0.4064
  circle A261 centre (17.67, 60.315) radius 0.75
  circle A262 centre (19.47, 58.915) radius 0.4064
  circle A263 centre (11.7, 68.6) radius 0.254
  circle A264 centre (12.455, 70.83) radius 0.4064
  circle A265 centre (11.055, 72.63) radius 0.75
  circle A266 centre (13.1, 67.2) radius 0.254
  circle A267 centre (14.7, 68.1) radius 0.254
  circle A268 centre (14.995, 70.83) radius 0.4064
  circle A269 centre (17.535, 70.83) radius 0.4064
  circle A270 centre (13.725, 73.37) radius 0.4064
  circle A271 centre (16.265, 73.37) radius 0.4064
  circle A272 centre (18.805, 73.37) radius 0.4064
  circle A273 centre (20.075, 70.83) radius 0.4064
  circle A274 centre (23.03, 70.23) radius 0.254
  circle A275 centre (21.345, 73.37) radius 0.4064
  circle A276 centre (24.5, 72.5) radius 0.254
  circle A277 centre (26.8, 57.4) radius 0.254
  circle A278 centre (29.3, 57.4) radius 0.254
  circle A279 centre (30.4, 58.3) radius 0.254
  circle A280 centre (28.9, 60) radius 0.254
  circle A281 centre (31.6, 59.4) radius 0.254
  circle A282 centre (32.2, 57.4) radius 0.254
  circle A283 centre (36.5, 57.8) radius 0.254
  circle A284 centre (30, 65.2) radius 0.254
  circle A285 centre (34.6, 64.8) radius 0.254
  circle A286 centre (37, 64.9) radius 0.254
  circle A287 centre (42.8, 57) radius 0.254
  circle A288 centre (41.5, 57.7) radius 0.254
  circle A289 centre (41.2, 60) radius 0.254
  circle A290 centre (43.5, 60.4) radius 0.254
  circle A291 centre (45.1, 60.8) radius 0.254
  circle A292 centre (31, 67.1) radius 0.254
  circle A293 centre (29.86, 68.94) radius 0.254
  circle A294 centre (31.8, 68.1) radius 0.254
  circle A295 centre (31.4, 70.3) radius 0.254
  circle A296 centre (32.9, 70.3) radius 0.254
  circle A297 centre (34.6, 72) radius 0.254
  circle A298 centre (31.8, 73.1) radius 0.254
  circle A299 centre (40.6, 65.4) radius 0.254
  circle A300 centre (46.4, 66.7) radius 0.254
  circle A301 centre (48.3, 65.6) radius 0.254
  circle A302 centre (42, 72.7) radius 0.254
  circle A303 centre (61.3, 43.4) radius 0.254
  circle A304 centre (59.2, 45.4) radius 0.254
  circle A305 centre (60.3, 44.5) radius 0.254
  circle A306 centre (58.4, 46.9) radius 0.254
  circle A307 centre (62.4, 47.4) radius 0.254
  circle A308 centre (71.9, 41.7) radius 0.254
  circle A309 centre (70.6, 42.4) radius 0.254
  circle A310 centre (75.2, 44) radius 0.254
  circle A311 centre (71.8, 46.1) radius 0.254
  circle A312 centre (74.2, 47.9) radius 0.254
  circle A313 centre (59, 51) radius 0.254
  circle A314 centre (52.4, 53.6) radius 0.254
  circle A315 centre (52.1, 55.5) radius 0.254
  circle A316 centre (52.9, 56.8) radius 0.254
  circle A317 centre (60.2, 55.087) radius 0.4064
  circle A318 centre (67.7, 48.9) radius 0.254
  circle A319 centre (70, 50.1) radius 0.254
  circle A320 centre (97.8, 48.7) radius 0.254
  circle A321 centre (95.9, 49.8) radius 0.254
  circle A322 centre (98.315, 52.6854) radius 0.4064
  circle A323 centre (101.1281, 52.2968) radius 0.4064
  circle A324 centre (100.3137, 54.7027) radius 0.4064
  circle A325 centre (97.5006, 55.0913) radius 0.4064
  circle A326 centre (51.8, 60.7) radius 0.254
  circle A327 centre (60.2, 59.913) radius 0.4064
  circle A328 centre (50.9, 61.6) radius 0.254
  circle A329 centre (55.6, 63.3) radius 0.254
  circle A330 centre (55.6, 64.7) radius 0.254
  circle A331 centre (58.2, 64.5) radius 0.254
  circle A332 centre (65.6, 60.7) radius 0.254
  circle A333 centre (55.8, 66.5) radius 0.254
  circle A334 centre (54.6, 67.8) radius 0.254
  circle A335 centre (61, 69.2) radius 0.254
  circle A336 centre (52.925, 70.53) radius 0.4064
  circle A337 centre (55.465, 70.53) radius 0.4064
  circle A338 centre (51.1, 72.8) radius 0.254
  circle A339 centre (54.195, 73.07) radius 0.4064
  circle A340 centre (56.735, 73.07) radius 0.4064
  circle A341 centre (58.005, 70.53) radius 0.4064
  circle A342 centre (60.675, 71.27) radius 0.75
  circle A343 centre (59.275, 73.07) radius 0.4064
  circle A344 centre (67.9, 73.5) radius 0.254
  circle A345 centre (72.495, 70.33) radius 0.4064
  circle A346 centre (75.035, 70.33) radius 0.4064
  circle A347 centre (73.765, 72.87) radius 0.4064
  circle A348 centre (96.6863, 57.4973) radius 0.4064
  circle A349 centre (99.4994, 57.1087) radius 0.4064
  circle A350 centre (95.8719, 59.9032) radius 0.4064
  circle A351 centre (98.685, 59.5146) radius 0.4064
  circle A352 centre (77.705, 71.07) radius 0.75
  circle A353 centre (80.755, 70.33) radius 0.4064
  circle A354 centre (76.305, 72.87) radius 0.4064
  circle A355 centre (82.025, 72.87) radius 0.4064
  circle A356 centre (83.295, 70.33) radius 0.4064
  circle A357 centre (85.835, 70.33) radius 0.4064
  circle A358 centre (88.375, 70.33) radius 0.4064
  circle A359 centre (84.565, 72.87) radius 0.4064
  circle A360 centre (87.105, 72.87) radius 0.4064
  circle A361 centre (91.045, 71.07) radius 0.75
  circle A362 centre (89.645, 72.87) radius 0.4064
extrude "Extrusion2" add sketch "Skizze6 outline for Extrusion2" along normal blind 2
